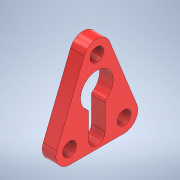
# Autodesk Inventor part: Part3
Saved by Autodesk Inventor 2021 (Build 250183000, 183)
## iProperties
Created: 2022-04-24
Part Number: Part3
Material: Generic
Document SubType Name: Modeling
Designer: hp
Density: 1 g/cm^3
Appearance: Light Red
Author: hp
Autodesk Inventor part; units mm, degrees
ref_plane "YZ Plane" through (0, 0, 0) normal (1, 0, 0) x (0, 1, 0)
ref_plane "XZ Plane" through (0, 0, 0) normal (0, 1, 0) x (-1, 0, 0)
ref_plane "XY Plane" through (0, 0, 0) normal (0, 0, 1) x (1, 0, 0)
sketch "Sketch1" plane through (0, 0, 0) normal (0, 1, 0) x (-1, 0, 0)
  point P0 (0, 0)
extrude "Extrusion1" [suppressed]
sketch "Sketch2" plane through (0, 0, 0) normal (1, 0, 0) x (0, 1, 0)
  arc A0 (-9.8478, -6.8571) -> (-9.8478, 6.8571) centre (0, 0) ccw
  line L0 (0, 0) -> (-30, 0)
  arc A1 (-30, 6) -> (-30, -6) centre (-30, 0) ccw
  line L1 (-30, -6) -> (-11.4891, -6)
  line L2 (-30, 6) -> (-11.4891, 6)
  arc A2 (-9.8478, -6.8571) -> (-11.4891, -6) centre (-11.4891, -8) ccw
  arc A3 (-11.4891, 6) -> (-9.8478, 6.8571) centre (-11.4891, 8) ccw
  line L3 (0, 0) -> (-28, 0)
  line L4 (-28, 0) -> (-28, -20)
  line L5 (-28, -20) -> (-28, 20)
  circle A4 centre (-28, -20) radius 5
  circle A5 centre (-28, 20) radius 5
  line L6 (0, 0) -> (22, 0)
  circle A6 centre (22, 0) radius 5
  circle A7 centre (22, 0) radius 10
  circle A8 centre (-28, -20) radius 10
  circle A9 centre (-28, 20) radius 10
  line L7 (25.7139, -9.2848) -> (-24.2861, -29.2848)
  line L8 (-38, -20) -> (-38, 20)
  line L9 (-24.2861, 29.2848) -> (25.7139, 9.2848)
  point P0 (-10.3923, -6)
  point P1 (-10.3923, 6)
  dimension "d15" = 24
  dimension "d16" = 30
  dimension "d17" = 12
  dimension "d18" = 2
  dimension "d19" = 28
  dimension "d20" = 20
  dimension "d21" = 40
  dimension "d22" = 10
  dimension "d23" = 10
  dimension "d24" = 22
  dimension "d25" = 10
  dimension "d26" = 20
  dimension "d27" = 20
  dimension "d28" = 20
  constraints: 20 end point, 16 point on circle, 12 tangent, 10 centre point, 8 coincident, 4 point on line, 3 horizontal, 1 equal radius, 1 parallel, 1 perpendicular
  measures "d15" diameter of A0
  measures "d16" distance of L0.start L0.end
  measures "d17" diameter of A1
  measures "d18" radius of A2
  measures "d19" distance of L0.start L3.end
  measures "d20" distance of L3.end L4.end
  measures "d21" distance of L4.end L5.end
  measures "d22" diameter of A4
  measures "d23" diameter of A5
  measures "d24" distance of L0.start L6.end
  measures "d25" diameter of A6
  measures "d26" diameter of A7
  measures "d27" diameter of A8
  measures "d28" diameter of A9
extrude "Extrusion2" add sketch "Sketch2" along normal blind 10 contours A0 A7 L7 A8 L4 L1 A2 | A0 A3 L2 L5 A9 L9 A7 | A7 | L4 A8 L8 A9 L5 L2 A1 L1 | A9 | A8
equation "\"d10\" = 0.5 * d9"
equation "\"d9\" = 6"
body "Solid1"
